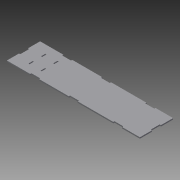
# Autodesk Inventor part: lado1
Saved by Autodesk Inventor 2015 (Build 190159000, 159)
## iProperties
Created: 2017-09-28
Part Number: lado1
Material: Generic
Document SubType Name: Modeling
Designer: Max
Density: 1 g/cm^3
Appearance: Default
Author: Max
Autodesk Inventor part; units mm, degrees
ref_plane "YZ Plane" through (0, 0, 0) normal (1, 0, 0) x (0, 1, 0)
ref_plane "XZ Plane" through (0, 0, 0) normal (0, 1, 0) x (-1, 0, 0)
ref_plane "XY Plane" through (0, 0, 0) normal (0, 0, 1) x (1, 0, 0)
sketch "Sketch1" plane through (0, 0, 0) normal (0, 0, 1) x (1, 0, 0)
  line L0 (-280, 0) -> (-280, 5.5)
  line L1 (-280, 5.5) -> (-320, 5.5)
  line L2 (-320, 5.5) -> (-320, 0)
  line L3 (-80, 0) -> (-80, 5.5)
  line L4 (-80, 5.5) -> (-120, 5.5)
  line L5 (-120, 5.5) -> (-120, 0)
  line L6 (-280, 150) -> (-280, 144.5)
  line L7 (-280, 144.5) -> (-320, 144.5)
  line L8 (-320, 144.5) -> (-320, 150)
  line L9 (-80, 150) -> (-80, 144.5)
  line L10 (-80, 144.5) -> (-120, 144.5)
  line L11 (-120, 144.5) -> (-120, 150)
  line L12 (-455, 0) -> (-455, 5.5)
  line L13 (-455, 5.5) -> (-495, 5.5)
  line L14 (-495, 5.5) -> (-495, 0)
  line L15 (-455, 150) -> (-455, 144.5)
  line L16 (-455, 144.5) -> (-495, 144.5)
  line L17 (-495, 144.5) -> (-495, 150)
  line L18 (-600, 55) -> (-594.5, 55)
  line L19 (-594.5, 55) -> (-594.5, 95)
  line L20 (-594.5, 95) -> (-600, 95)
  line L21 (0, 55) -> (-5.5, 55)
  line L22 (-5.5, 55) -> (-5.5, 95)
  line L23 (-5.5, 95) -> (0, 95)
  line L24 (-495, 150) -> (-600, 150)
  line L25 (-455, 150) -> (-320, 150)
  line L26 (-280, 150) -> (-120, 150)
  line L27 (-80, 150) -> (0, 150)
  line L28 (0, 0) -> (-80, 0)
  line L29 (-120, 0) -> (-280, 0)
  line L30 (-320, 0) -> (-455, 0)
  line L31 (-495, 0) -> (-600, 0)
  line L32 (0, 150) -> (0, 95)
  line L33 (0, 55) -> (0, 0)
  line L34 (-600, 150) -> (-600, 95)
  line L35 (-600, 55) -> (-600, 0)
  dimension "d0" = 600
  dimension "d1" = 150
  dimension "d4" = 40
  dimension "d5" = 5.5
  dimension "d8" = 40
  dimension "d9" = 5.5
  dimension "d10" = 40
  dimension "d11" = 5.5
  dimension "d12" = 40
  dimension "d13" = 5.5
  dimension "d14" = 40
  dimension "d15" = 5.5
  dimension "d17" = 5.5
  dimension "d18" = 40
  dimension "d19" = 5.5
  dimension "d23" = 480
  constraints: 72 end point, 10 parallel, 5 horizontal, 4 collinear, 3 vertical, 2 perpendicular
  measures "d0" distance of L24.end L27.end
  measures "d1" distance of L31.end L24.end
  measures "d4" distance of L1.end L0.end
  measures "d5" distance of L0.end L0.start
  measures "d8" distance of L4.end L3.end
  measures "d9" distance of L3.end L3.start
  measures "d10" distance of L6.end L7.end
  measures "d11" distance of L6.start L6.end
  measures "d12" distance of L9.end L10.end
  measures "d13" distance of L9.start L9.end
  measures "d14" distance of L13.end L12.end
  measures "d15" distance of L12.end L12.start
  measures "d17" distance of L20.end L19.end
  measures "d18" distance of L19.end L18.end
  measures "d19" distance of L22.end L23.end
  measures "d23" distance from line of L35 L4.end
extrude "Extrusion1" add sketch "Sketch1" along normal blind 5.5
sketch "Sketch2" plane through (0, 0, 5.5) normal (0, 0, 1) x (1, 0, 0)
  line L0 (-539.343, 36.6) -> (-534.3429, 36.6)
  line L1 (-534.3429, 36.6) -> (-534.3429, 56.6)
  line L2 (-534.3429, 56.6) -> (-539.343, 56.6)
  line L3 (-539.343, 56.6) -> (-539.343, 36.6)
  line L4 (-539.343, 93.3) -> (-534.343, 93.3)
  line L5 (-534.343, 93.3) -> (-534.343, 113.3)
  line L6 (-534.343, 113.3) -> (-539.343, 113.3)
  line L7 (-539.343, 113.3) -> (-539.343, 93.3)
  line L8 (-484.3429, 113.3) -> (-479.3429, 113.3)
  line L9 (-479.3429, 113.3) -> (-479.3429, 93.3)
  line L10 (-479.3429, 93.3) -> (-484.3429, 93.3)
  line L11 (-484.3429, 93.3) -> (-484.3429, 113.3)
  line L12 (-479.3429, 56.6) -> (-484.3429, 56.6)
  line L13 (-484.3429, 56.6) -> (-484.3429, 36.6)
  line L14 (-484.3429, 36.6) -> (-479.3429, 36.6)
  line L15 (-479.3429, 36.6) -> (-479.3429, 56.6)
  line L16 (-600, 150) -> (-600, 95) projected
  point P0 (0, 0)
  dimension "d26" = 20
  dimension "d27" = 5
  dimension "d28" = 20
  dimension "d29" = 5
  dimension "d30" = 20
  dimension "d33" = 60.657
  constraints: 32 end point, 8 parallel, 4 horizontal, 4 perpendicular, 3 point on line
  measures "d26" distance of L1.end L0.end
  measures "d27" distance of L6.end L5.end
  measures "d28" distance of L5.end L4.end
  measures "d29" distance of L9.end L10.end
  measures "d30" distance of L8.end L9.end
  measures "d33" distance between parallel lines of L16 L7
extrude "Extrusion2" cut sketch "Sketch2" against normal blind 10
body "Solid1"
